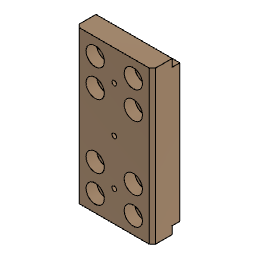
Spindle mount support (Autodesk Fusion 360 design; units mm, degrees)
Autodesk Fusion 360 part; units mm, degrees
sketch "Board" plane through (0, 0, 0) normal (0, 1, 0) x (1, 0, 0)
  line L0 (-25, -45) -> (-25, -50)
  circle A0 centre (12.5, -39) radius 6
  line L1 (-25, -50) -> (25, -50)
  circle A1 centre (12.5, -21) radius 2.5
  circle A2 centre (12.5, 21) radius 2.5
  line L2 (-25, 50) -> (25, 50)
  circle A3 centre (0, 30) radius 1.5
  line L3 (-25, 45) -> (-25, 50)
  circle A4 centre (12.5, 39) radius 6
  circle A5 centre (-12.5, 21) radius 2.5
  circle A6 centre (12.5, 21) radius 6
  line L4 (25, 50) -> (25, 45)
  circle A7 centre (12.5, -21) radius 6
  line L5 (-25, 50) -> (25, 50)
  circle A8 centre (-12.5, 21) radius 6
  circle A9 centre (-12.5, -21) radius 2.5
  line L6 (25, 50) -> (-25, 50)
  circle A10 centre (12.5, 39) radius 2.5
  circle A11 centre (-12.5, 39) radius 6
  circle A12 centre (-12.5, 39) radius 2.5
  line L7 (25, -45) -> (-25, -45)
  line L8 (25, -50) -> (-25, -50)
  circle A13 centre (12.5, -39) radius 2.5
  circle A14 centre (-12.5, -39) radius 6
  circle A15 centre (0, -30) radius 1.5
  circle A16 centre (-12.5, -39) radius 2.5
  line L9 (25, -50) -> (25, -45)
  line L10 (25, 50) -> (25, -50)
  line L11 (25, 45) -> (-25, 45)
  line L12 (-25, -50) -> (-25, 50)
  circle A17 centre (0, 0) radius 1.5
  circle A18 centre (-12.5, -21) radius 6
  dimension "d23" = 100
  dimension "d24" = 5
  dimension "d25" = 5
  dimension "d26" = 5
  dimension "d27" = 5
  dimension "d28" = 5
  dimension "d29" = 5
  dimension "d30" = 5
  dimension "d31" = 5
  dimension "d32" = 3
  dimension "d33" = 3
  dimension "d34" = 3
  dimension "d35" = 12
  dimension "d36" = 12
  dimension "d37" = 12
  dimension "d38" = 12
  dimension "d39" = 12
  dimension "d40" = 12
  dimension "d41" = 12
  dimension "d42" = 12
  dimension "d43" = 5
  dimension "d44" = 5
  constraint horizontal L2
  constraint vertical L10
  constraint horizontal L8
  constraint vertical L12
  constraint coincident L2.start L3.end
  constraint concentric A5 A8
  constraint horizontal L5
  constraint vertical L4
  constraint horizontal L11
  constraint vertical L3
  constraint horizontal L1
  constraint vertical L9
  constraint horizontal L7
  constraint vertical L0
  measures "d23" distance of L2.start L0.end
  measures "d24" diameter of A12
  measures "d25" diameter of A10
  measures "d26" diameter of A5
  measures "d27" diameter of A2
  measures "d28" diameter of A9
  measures "d29" diameter of A1
  measures "d30" diameter of A16
  measures "d31" diameter of A13
  measures "d32" diameter of A15
  measures "d33" diameter of A17
  measures "d34" diameter of A3
  measures "d35" diameter of A11
  measures "d36" diameter of A4
  measures "d37" diameter of A8
  measures "d38" diameter of A6
  measures "d39" diameter of A18
  measures "d40" diameter of A7
  measures "d41" diameter of A14
  measures "d42" diameter of A0
  measures "d43" distance of L3.start L2.start
  measures "d44" distance of L0.end L0.start
extrude "Extrude1" add sketch "Board" along normal blind 13 contours L0 L1 L7 L8 L9 L10 L12 | L2 L3 L4 L5 L6 L10 L11 L12 makes body 1 at (8.3333, 4.3333, 45) makes body 2 at (-8.3333, 4.3333, -50)
extrude "Extrude2" add sketch "Board" along normal blind 18 contours A14 | A0 | A4 | A11 | L7 L10 L11 L12 | A3 | A6 | A7 | A8 | A15 | A17 | A18 bodies 1 2
extrude "Extrude3" cut sketch "Board" along normal blind 7 contours A14 | A0 | A4 | A11 | A6 | A7 | A8 | A18 bodies 1
extrude "Extrude4" cut sketch "Board" along normal blind 7 contours A3 | A15 | A17 bodies 1
chamfer "Chamfer1" distance 2 angle 45 2 edges at (25, 0, 0) (-25, 0, 0) on bodies 1
named bodies: "Board"
